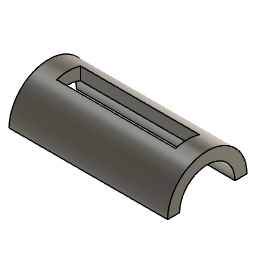
protipo2_SimilarACuero v1 (Autodesk Fusion 360 design; units mm, degrees)
Autodesk Fusion 360 part; units mm, degrees
sketch "Boceto1" plane through (0, 0, 0) normal (1, 0, 0) x (0, 1, 0)
sketch "Boceto2" plane through (0, 0, 0) normal (1, 0, 0) x (0, 1, 0)
  line L0 (-50, 0) -> (-35, 0)
  line L1 (35, 0) -> (50, 0)
  arc A0 (50, 0) -> (-50, 0) centre (0, 0) ccw
  arc A1 (35, 0) -> (-35, 0) centre (0, 0) ccw
  dimension "d1" = 100
  dimension "d2" = 15
  constraint coincident A0.centre A1.centre
  constraint horizontal L0
  constraint horizontal L0.start A0.centre
  constraint horizontal L1
  constraint horizontal A0.centre L1.start
  measures "d1" diameter of A0
  measures "d2" distance of L0.start L0.end
extrude "Extruir1" add sketch "Boceto2" along normal blind 200
ref_plane "PlanoDeObra1" through (100, 0, 50) normal (0, 0, 1) x (0, -1, 0)
sketch "Boceto3" plane through (100, 0, 50) normal (0, 0, 1) x (1, 0, 0)
  line L0 (75, -15) -> (-75, -15)
  line L1 (-75, -15) -> (-75, 15)
  line L2 (-75, 15) -> (75, 15)
  line L3 (75, 15) -> (75, -15)
  line L4 (75, -15) -> (-75, 15) construction
  line L5 (-75, -15) -> (75, 15) construction
  dimension "d6" = 150
  dimension "d7" = 30
  constraint horizontal L0
  constraint perpendicular L0 L1
  constraint parallel L0 L2
  constraint parallel L1 L3
  constraint coincident L4 origin
  constraint coincident L5 origin
  measures "d6" distance of L1.end L2.end
  measures "d7" distance of L0.end L1.end
extrude "Extruir2" cut sketch "Boceto3" along normal up to surface end surface at (66.6667, -26.8116, 22.4976)
sketch "Boceto4" plane through (0, 0, 0) normal (0, 0, 1) x (1, 0, 0)
